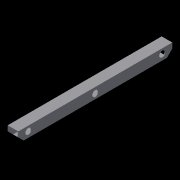
# Autodesk Inventor part: Side Box Tube
Saved by Autodesk Inventor 2014 SP1 (Build 180222100, 222)
## iProperties
Created: 2013-11-29
Part Number: Side Box Tube
Material: Generic
Document SubType Name: Modeling
Designer: Rauhul Varma
Mass: 422.488 g
Surface Area: 2692.85 cm^2
Volume: 422.488 cm^3
Density: 1 g/cm^3
Appearance: Default
Author: Rauhul Varma
Autodesk Inventor part; units mm, degrees
ref_plane "YZ Plane" through (0, 0, 0) normal (1, 0, 0) x (0, 1, 0)
ref_plane "XZ Plane" through (0, 0, 0) normal (0, 1, 0) x (-1, 0, 0)
ref_plane "XY Plane" through (0, 0, 0) normal (0, 0, 1) x (1, 0, 0)
sketch "Sketch1" plane through (0, 0, 0) normal (0, 0, 1) x (1, 0, 0)
  line L0 (0, 0) -> (50.8, 0)
  line L1 (50.8, 0) -> (50.8, 50.8)
  line L2 (50.8, 50.8) -> (0, 50.8)
  line L3 (0, 50.8) -> (0, 0)
  line L4 (3.175, 3.175) -> (47.625, 3.175)
  line L5 (47.625, 3.175) -> (47.625, 47.625)
  line L6 (47.625, 47.625) -> (3.175, 47.625)
  line L7 (3.175, 47.625) -> (3.175, 3.175)
  dimension "d0" = 50.8
  dimension "d1" = 50.8
  dimension "d2" = 3.175
  dimension "d3" = 3.175
  dimension "d4" = 3.175
  dimension "d5" = 3.175
  constraints: 16 end point, 4 parallel, 2 horizontal, 2 perpendicular
  measures "d0" distance of L2.end L1.end
  measures "d1" distance of L1.end L0.end
  measures "d2" distance between parallel lines of L2 L6
  measures "d3" distance between parallel lines of L1 L5
  measures "d4" distance between parallel lines of L0 L4
  measures "d5" distance between parallel lines of L3 L7
extrude "Box Beam Profile" add sketch "Sketch1" along normal blind 736.6
sketch "Sketch2" plane through (0, 0, 0) normal (-1, 0, 0) x (0, 0, 1)
  line L0 (0, 50.8) -> (0, 0) projected
  line L1 (0, 0) -> (736.6, 0) projected
  line L2 (736.6, 50.8) -> (736.6, 0) projected
  line L3 (0, 50.8) -> (736.6, 50.8) projected
  line L4 (0, 25.4) -> (25.4, 0)
  line L5 (0, 25.4) -> (736.6, 25.4) construction
  line L6 (368.3, 50.8) -> (368.3, 0) construction
  circle A0 centre (368.3, 23.8125) radius 14.2875
  line L7 (736.6, 25.4) -> (711.2, 0)
  circle A1 centre (48.0396, 26.9875) radius 14.2875
  circle A2 centre (688.5604, 26.9875) radius 14.2875
  line L8 (0, 25.4) -> (25.4, 25.4)
  line L9 (25.4, 50.8) -> (25.4, 25.4)
  line L10 (736.6, 25.4) -> (711.2, 25.4)
  line L11 (711.2, 50.8) -> (711.2, 25.4)
  line L12 (368.4416, 9.5257) -> (688.702, 12.7007) construction
  line L13 (688.4188, 41.2743) -> (368.1584, 38.0993) construction
  line L14 (368.4416, 38.0993) -> (48.1812, 41.2743) construction
  line L15 (47.898, 12.7007) -> (368.1584, 9.5257) construction
  dimension "d8" = 45
  dimension "d9" = 28.575
  dimension "d10" = 45
  dimension "d11" = 320.2761
  dimension "d12" = 25.4
  dimension "d13" = 25.4
  dimension "d16" = 1.5875
  dimension "d17" = 1.5875
  dimension "d18" = 1.5875
  constraints: 24 end point, 8 point on circle, 8 tangent, 7 point on line, 4 midpoint, 3 centre point, 3 perpendicular, 2 equal radius, 1 symmetric about line
  measures "d8" angle of L0 L4
  measures "d9" diameter of A0
  measures "d10" angle of L2 L7
  measures "d11" distance of A2.centre A0.centre
  measures "d12" distance between parallel lines of L0 L9
  measures "d13" distance between parallel lines of L2 L11
  measures "d16" distance from line of L5 A0.centre
  measures "d17" distance from line of L5 A2.centre
  measures "d18" distance from line of L5 A1.centre
extrude "Through Cutouts" cut sketch "Sketch2" against normal through all contours L4 L1 L0 | L7 L2 L1 | A0 | A1 | A2
body "Solid1"
